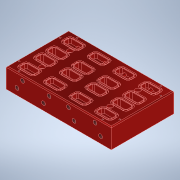
# Autodesk Inventor part: UNLHEP-14-01-P-004_ChuckForGantry
Saved by Autodesk Inventor 2022 (Build 260153000, 153)
## iProperties
Created: 2014-01-09
Part Number: UNLHEP-14-01-P-004_ChuckForGantry
Material: Aluminum, Anodized Red
Document SubType Name: Modeling
Designer: Frank Meier
Density: 2.7 g/cm^3
Project: UNL Pixel Phase I
Mass: 2699.72 g
Surface Area: 1115.91 cm^2
Volume: 999.896 cm^3
Appearance: Anodized - Red
Author: Frank Meier
Revision Number: 00
Autodesk Inventor part; units mm, degrees
ref_plane "YZ Plane" through (0, 0, 0) normal (1, 0, 0) x (0, 1, 0)
ref_plane "XZ Plane" through (0, 0, 0) normal (0, 1, 0) x (-1, 0, 0)
ref_plane "XY Plane" through (0, 0, 0) normal (0, 0, 1) x (1, 0, 0)
sketch "Skizze1" plane through (0, 0, 0) normal (0, 0, 1) x (1, 0, 0)
  line L0 (-117.475, -69.85) -> (117.475, -69.85)
  line L1 (117.475, -69.85) -> (117.475, 69.85)
  line L2 (117.475, 69.85) -> (-117.475, 69.85)
  line L3 (-117.475, 69.85) -> (-117.475, -69.85)
  line L4 (-117.475, -69.85) -> (117.475, 69.85) construction
  line L5 (117.475, -69.85) -> (-117.475, 69.85) construction
  point P0 (0, 0)
  dimension "d0" = 234.95
  dimension "d2" = 139.7
  constraints: 12 end point, 2 midpoint, 2 parallel, 1 horizontal, 1 perpendicular
  measures "d0" distance of L1.end L2.end
  measures "d2" distance of L0.end L1.end
extrude "Extrusion1" add sketch "Skizze1" along normal blind 44.45
chamfer "Fase1" distance 2 angle 45 4 edges at (0, -69.85, 44.45) (-117.475, 0, 44.45) (0, 69.85, 44.45) (117.475, 0, 44.45)
sketch "Alignment Holes" plane through (0, 0, 44.45) normal (0, 0, 1) x (1, 0, 0)
  line L0 (117.475, 69.85) -> (-117.475, 69.85) projected
  line L1 (117.475, -69.85) -> (117.475, 69.85) projected
  line L2 (-117.475, 69.85) -> (-117.475, -69.85) projected
  line L3 (-117.475, -69.85) -> (117.475, -69.85) projected
  point P0 (-112.475, 45.85)
  point P1 (-112.475, -45.85)
  point P2 (-93.475, -64.85)
  point P3 (-93.475, 64.85)
  point P4 (93.475, 64.85)
  point P5 (112.475, 45.85)
  point P6 (112.475, -45.85)
  point P7 (93.475, -64.85)
  dimension "d153" = 24
  dimension "d154" = 24
  dimension "d155" = 5
  dimension "d156" = 5
  dimension "d157" = 24
  dimension "d158" = 5
  dimension "d159" = 5
  dimension "d160" = 24
  dimension "d161" = 24
  dimension "d162" = 5
  dimension "d163" = 5
  dimension "d164" = 24
  dimension "d165" = 5
  dimension "d166" = 24
  dimension "d167" = 5
  dimension "d168" = 24
  measures "d153" distance from line of L0 point (-112.475, 45.85)
  measures "d154" distance from line of L3 point (-112.475, -45.85)
  measures "d155" distance from line of L2 point (-112.475, -45.85)
  measures "d156" distance from line of L3 point (-93.475, -64.85)
  measures "d157" distance from line of L2 point (-93.475, -64.85)
  measures "d158" distance from line of L2 point (-112.475, 45.85)
  measures "d159" distance from line of L0 point (-93.475, 64.85)
  measures "d160" distance from line of L2 point (-93.475, 64.85)
  measures "d161" distance from line of L1 point (93.475, 64.85)
  measures "d162" distance from line of L0 point (93.475, 64.85)
  measures "d163" distance from line of L1 point (112.475, 45.85)
  measures "d164" distance from line of L0 point (112.475, 45.85)
  measures "d165" distance from line of L1 point (112.475, -45.85)
  measures "d166" distance from line of L3 point (112.475, -45.85)
  measures "d167" distance from line of L3 point (93.475, -64.85)
  measures "d168" distance from line of L1 point (93.475, -64.85)
hole "Bohrung7" at (-112.475, 45.85, 44.45) at (-112.475, -45.85, 44.45) at (-93.475, -64.85, 44.45) at (-93.475, 64.85, 44.45) at (93.475, 64.85, 44.45) at (112.475, 45.85, 44.45) at (112.475, -45.85, 44.45) at (93.475, -64.85, 44.45) direction (0, 0, -1) diameter 3.242 depth 20 tip angle 118 thread size "M4x0.7" class "6H" standard "ISO Metric profile"
sketch "Wells" plane through (0, 0, 44.45) normal (0, 0, 1) x (1, 0, 0)
  line L0 (-97.975, 56.35) -> (-73.975, 56.35)
  line L1 (-70.975, 53.35) -> (-70.975, 44.35)
  line L2 (-73.975, 41.35) -> (-97.975, 41.35)
  line L3 (-100.975, 44.35) -> (-100.975, 53.35)
  circle A0 centre (-93.475, 64.85) radius 1.621 projected
  circle A1 centre (-112.475, 45.85) radius 1.621 projected
  arc A2 (-97.975, 56.35) -> (-100.975, 53.35) centre (-97.975, 53.35) ccw
  arc A3 (-70.975, 53.35) -> (-73.975, 56.35) centre (-73.975, 53.35) ccw
  arc A4 (-73.975, 41.35) -> (-70.975, 44.35) centre (-73.975, 44.35) ccw
  arc A5 (-100.975, 44.35) -> (-97.975, 41.35) centre (-97.975, 44.35) ccw
  arc A6 (-40.658, 56.35) -> (-43.658, 53.35) centre (-40.658, 53.35) ccw
  line L4 (-43.658, 44.35) -> (-43.658, 53.35)
  arc A7 (-43.658, 44.35) -> (-40.658, 41.35) centre (-40.658, 44.35) ccw
  line L5 (-40.658, 56.35) -> (-16.658, 56.35)
  arc A8 (-13.658, 53.35) -> (-16.658, 56.35) centre (-16.658, 53.35) ccw
  line L6 (-13.658, 53.35) -> (-13.658, 44.35)
  line L7 (-16.658, 41.35) -> (-40.658, 41.35)
  arc A9 (-16.658, 41.35) -> (-13.658, 44.35) centre (-16.658, 44.35) ccw
  arc A10 (16.659, 56.35) -> (13.659, 53.35) centre (16.659, 53.35) ccw
  line L8 (13.659, 44.35) -> (13.659, 53.35)
  arc A11 (13.659, 44.35) -> (16.659, 41.35) centre (16.659, 44.35) ccw
  line L9 (16.659, 56.35) -> (40.659, 56.35)
  arc A12 (43.659, 53.35) -> (40.659, 56.35) centre (40.659, 53.35) ccw
  line L10 (43.659, 53.35) -> (43.659, 44.35)
  line L11 (40.659, 41.35) -> (16.659, 41.35)
  arc A13 (40.659, 41.35) -> (43.659, 44.35) centre (40.659, 44.35) ccw
  arc A14 (73.976, 56.35) -> (70.976, 53.35) centre (73.976, 53.35) ccw
  line L12 (70.976, 44.35) -> (70.976, 53.35)
  arc A15 (70.976, 44.35) -> (73.976, 41.35) centre (73.976, 44.35) ccw
  line L13 (73.976, 56.35) -> (97.976, 56.35)
  arc A16 (100.976, 53.35) -> (97.976, 56.35) centre (97.976, 53.35) ccw
  line L14 (100.976, 53.35) -> (100.976, 44.35)
  line L15 (97.976, 41.35) -> (73.976, 41.35)
  arc A17 (97.976, 41.35) -> (100.976, 44.35) centre (97.976, 44.35) ccw
  arc A18 (-97.975, 20.784) -> (-100.975, 17.784) centre (-97.975, 17.784) ccw
  line L16 (-100.975, 8.784) -> (-100.975, 17.784)
  arc A19 (-100.975, 8.784) -> (-97.975, 5.784) centre (-97.975, 8.784) ccw
  line L17 (-97.975, 20.784) -> (-73.975, 20.784)
  arc A20 (-70.975, 17.784) -> (-73.975, 20.784) centre (-73.975, 17.784) ccw
  line L18 (-70.975, 17.784) -> (-70.975, 8.784)
  line L19 (-73.975, 5.784) -> (-97.975, 5.784)
  arc A21 (-73.975, 5.784) -> (-70.975, 8.784) centre (-73.975, 8.784) ccw
  arc A22 (-40.658, 20.784) -> (-43.658, 17.784) centre (-40.658, 17.784) ccw
  line L20 (-43.658, 8.784) -> (-43.658, 17.784)
  arc A23 (-43.658, 8.784) -> (-40.658, 5.784) centre (-40.658, 8.784) ccw
  line L21 (-40.658, 20.784) -> (-16.658, 20.784)
  arc A24 (-13.658, 17.784) -> (-16.658, 20.784) centre (-16.658, 17.784) ccw
  line L22 (-13.658, 17.784) -> (-13.658, 8.784)
  line L23 (-16.658, 5.784) -> (-40.658, 5.784)
  arc A25 (-16.658, 5.784) -> (-13.658, 8.784) centre (-16.658, 8.784) ccw
  arc A26 (16.659, 20.784) -> (13.659, 17.784) centre (16.659, 17.784) ccw
  line L24 (13.659, 8.784) -> (13.659, 17.784)
  arc A27 (13.659, 8.784) -> (16.659, 5.784) centre (16.659, 8.784) ccw
  line L25 (16.659, 20.784) -> (40.659, 20.784)
  arc A28 (43.659, 17.784) -> (40.659, 20.784) centre (40.659, 17.784) ccw
  line L26 (43.659, 17.784) -> (43.659, 8.784)
  line L27 (40.659, 5.784) -> (16.659, 5.784)
  arc A29 (40.659, 5.784) -> (43.659, 8.784) centre (40.659, 8.784) ccw
  arc A30 (73.976, 20.784) -> (70.976, 17.784) centre (73.976, 17.784) ccw
  line L28 (70.976, 8.784) -> (70.976, 17.784)
  arc A31 (70.976, 8.784) -> (73.976, 5.784) centre (73.976, 8.784) ccw
  line L29 (73.976, 20.784) -> (97.976, 20.784)
  arc A32 (100.976, 17.784) -> (97.976, 20.784) centre (97.976, 17.784) ccw
  line L30 (100.976, 17.784) -> (100.976, 8.784)
  line L31 (97.976, 5.784) -> (73.976, 5.784)
  arc A33 (97.976, 5.784) -> (100.976, 8.784) centre (97.976, 8.784) ccw
  circle A34 centre (-93.475, -64.85) radius 1.621 projected
  circle A35 centre (112.475, 45.85) radius 1.621 projected
  line L32 (97.975, -56.35) -> (73.975, -56.35)
  line L33 (70.975, -53.35) -> (70.975, -44.35)
  line L34 (73.975, -41.35) -> (97.975, -41.35)
  line L35 (100.975, -44.35) -> (100.975, -53.35)
  circle A36 centre (112.475, -45.85) radius 1.621 projected
  circle A37 centre (93.475, -64.85) radius 1.621 projected
  arc A38 (73.975, -41.35) -> (70.975, -44.35) centre (73.975, -44.35) ccw
  arc A39 (70.975, -53.35) -> (73.975, -56.35) centre (73.975, -53.35) ccw
  arc A40 (97.975, -56.35) -> (100.975, -53.35) centre (97.975, -53.35) ccw
  arc A41 (100.975, -44.35) -> (97.975, -41.35) centre (97.975, -44.35) ccw
  arc A42 (43.658, -44.35) -> (40.658, -41.35) centre (40.658, -44.35) ccw
  line L36 (16.658, -41.35) -> (40.658, -41.35)
  line L37 (43.658, -44.35) -> (43.658, -53.35)
  arc A43 (40.658, -56.35) -> (43.658, -53.35) centre (40.658, -53.35) ccw
  line L38 (40.658, -56.35) -> (16.658, -56.35)
  arc A44 (16.658, -41.35) -> (13.658, -44.35) centre (16.658, -44.35) ccw
  arc A45 (13.658, -53.35) -> (16.658, -56.35) centre (16.658, -53.35) ccw
  line L39 (13.658, -53.35) -> (13.658, -44.35)
  arc A46 (-13.659, -44.35) -> (-16.659, -41.35) centre (-16.659, -44.35) ccw
  line L40 (-40.659, -41.35) -> (-16.659, -41.35)
  line L41 (-13.659, -44.35) -> (-13.659, -53.35)
  arc A47 (-16.659, -56.35) -> (-13.659, -53.35) centre (-16.659, -53.35) ccw
  line L42 (-16.659, -56.35) -> (-40.659, -56.35)
  arc A48 (-40.659, -41.35) -> (-43.659, -44.35) centre (-40.659, -44.35) ccw
  arc A49 (-43.659, -53.35) -> (-40.659, -56.35) centre (-40.659, -53.35) ccw
  line L43 (-43.659, -53.35) -> (-43.659, -44.35)
  arc A50 (-70.976, -44.35) -> (-73.976, -41.35) centre (-73.976, -44.35) ccw
  line L44 (-97.976, -41.35) -> (-73.976, -41.35)
  line L45 (-70.976, -44.35) -> (-70.976, -53.35)
  arc A51 (-73.976, -56.35) -> (-70.976, -53.35) centre (-73.976, -53.35) ccw
  line L46 (-73.976, -56.35) -> (-97.976, -56.35)
  arc A52 (-97.976, -41.35) -> (-100.976, -44.35) centre (-97.976, -44.35) ccw
  arc A53 (-100.976, -53.35) -> (-97.976, -56.35) centre (-97.976, -53.35) ccw
  line L47 (-100.976, -53.35) -> (-100.976, -44.35)
  arc A54 (100.975, -8.784) -> (97.975, -5.784) centre (97.975, -8.784) ccw
  line L48 (73.975, -5.784) -> (97.975, -5.784)
  line L49 (100.975, -8.784) -> (100.975, -17.784)
  arc A55 (97.975, -20.784) -> (100.975, -17.784) centre (97.975, -17.784) ccw
  line L50 (97.975, -20.784) -> (73.975, -20.784)
  arc A56 (73.975, -5.784) -> (70.975, -8.784) centre (73.975, -8.784) ccw
  arc A57 (70.975, -17.784) -> (73.975, -20.784) centre (73.975, -17.784) ccw
  line L51 (70.975, -17.784) -> (70.975, -8.784)
  arc A58 (43.658, -8.784) -> (40.658, -5.784) centre (40.658, -8.784) ccw
  line L52 (16.658, -5.784) -> (40.658, -5.784)
  line L53 (43.658, -8.784) -> (43.658, -17.784)
  arc A59 (40.658, -20.784) -> (43.658, -17.784) centre (40.658, -17.784) ccw
  line L54 (40.658, -20.784) -> (16.658, -20.784)
  arc A60 (16.658, -5.784) -> (13.658, -8.784) centre (16.658, -8.784) ccw
  arc A61 (13.658, -17.784) -> (16.658, -20.784) centre (16.658, -17.784) ccw
  line L55 (13.658, -17.784) -> (13.658, -8.784)
  arc A62 (-13.659, -8.784) -> (-16.659, -5.784) centre (-16.659, -8.784) ccw
  line L56 (-40.659, -5.784) -> (-16.659, -5.784)
  line L57 (-13.659, -8.784) -> (-13.659, -17.784)
  arc A63 (-16.659, -20.784) -> (-13.659, -17.784) centre (-16.659, -17.784) ccw
  line L58 (-16.659, -20.784) -> (-40.659, -20.784)
  arc A64 (-40.659, -5.784) -> (-43.659, -8.784) centre (-40.659, -8.784) ccw
  arc A65 (-43.659, -17.784) -> (-40.659, -20.784) centre (-40.659, -17.784) ccw
  line L59 (-43.659, -17.784) -> (-43.659, -8.784)
  arc A66 (-70.976, -8.784) -> (-73.976, -5.784) centre (-73.976, -8.784) ccw
  line L60 (-97.976, -5.784) -> (-73.976, -5.784)
  line L61 (-70.976, -8.784) -> (-70.976, -17.784)
  arc A67 (-73.976, -20.784) -> (-70.976, -17.784) centre (-73.976, -17.784) ccw
  line L62 (-73.976, -20.784) -> (-97.976, -20.784)
  arc A68 (-97.976, -5.784) -> (-100.976, -8.784) centre (-97.976, -8.784) ccw
  arc A69 (-100.976, -17.784) -> (-97.976, -20.784) centre (-97.976, -17.784) ccw
  line L63 (-100.976, -17.784) -> (-100.976, -8.784)
  point P0 (0, 0)
  point P1 (-70.975, 41.35)
  point P2 (-70.975, 56.35)
  point P3 (-100.975, 41.35)
  point P4 (-43.658, 41.35)
  point P5 (-13.658, 56.35)
  point P6 (-13.658, 41.35)
  point P7 (13.659, 41.35)
  point P8 (43.659, 56.35)
  point P9 (43.659, 41.35)
  point P10 (70.976, 41.35)
  point P11 (100.976, 56.35)
  point P12 (100.976, 41.35)
  point P13 (-100.975, 5.784)
  point P14 (-70.975, 20.784)
  point P15 (-70.975, 5.784)
  point P16 (-43.658, 5.784)
  point P17 (-13.658, 20.784)
  point P18 (-13.658, 5.784)
  point P19 (13.659, 5.784)
  point P20 (43.659, 20.784)
  point P21 (43.659, 5.784)
  point P22 (70.976, 5.784)
  point P23 (100.976, 20.784)
  point P24 (100.976, 5.784)
  point P25 (100.975, -56.35)
  point P26 (70.975, -56.35)
  point P27 (100.975, -41.35)
  point P28 (43.658, -41.35)
  point P29 (43.658, -56.35)
  point P30 (13.658, -56.35)
  point P31 (-13.659, -41.35)
  point P32 (-13.659, -56.35)
  point P33 (-43.659, -56.35)
  point P34 (-70.976, -41.35)
  point P35 (-70.976, -56.35)
  point P36 (-100.976, -56.35)
  point P37 (100.975, -5.784)
  point P38 (100.975, -20.784)
  point P39 (70.975, -20.784)
  point P40 (43.658, -5.784)
  point P41 (43.658, -20.784)
  point P42 (13.658, -20.784)
  point P43 (-13.659, -5.784)
  point P44 (-13.659, -20.784)
  point P45 (-43.659, -20.784)
  point P46 (-70.976, -5.784)
  point P47 (-70.976, -20.784)
  point P48 (-100.976, -20.784)
  dimension "d259" = 30
  dimension "d260" = 15
  dimension "d261" = 8.5
  dimension "d262" = 11.5
  dimension "d266" = 3
  dimension "d269" = 57.317
  dimension "d272" = 35.566
  dimension "d276" = 11.499
  dimension "d410" = 11.5
  dimension "d411" = 8.5
  dimension "d412" = 15
  dimension "d413" = 30
  dimension "d414" = 3
  dimension "d417" = 57.317
  dimension "d420" = 35.566
  constraints: 128 end point, 128 point on circle, 96 point on line, 64 centre point, 16 tangent, 6 equal radius, 4 collinear, 4 horizontal, 4 parallel, 2 perpendicular, 2 vertical, 318 other
  measures "d259" distance of point (-70.975, 41.35) point (-100.975, 41.35)
  measures "d260" distance of point (-70.975, 56.35) point (-70.975, 41.35)
  measures "d261" distance from line of L0 A0.centre
  measures "d262" distance from line of L3 A1.centre
  measures "d266" radius of A2
  measures "d269" distance of L3.end L4.end
  measures "d272" distance of L3.end L16.end
  measures "d276" distance from line of L14 A35.centre
  measures "d410" distance from line of L35 A36.centre
  measures "d411" distance from line of A37.centre L32
  measures "d412" distance of point (100.975, -41.35) point (100.975, -56.35)
  measures "d413" distance of point (100.975, -56.35) point (70.975, -56.35)
  measures "d414" radius of A38
  measures "d417" distance of point (100.975, -41.35) point (43.658, -41.35)
  measures "d420" distance of point (100.975, -41.35) point (100.975, -5.784)
extrude "Extrusion6" cut sketch "Wells" against normal blind 10 contours L0 A3 L1 A4 L2 A5 L3 A2 | L5 A8 L6 A9 L7 A7 L4 A6 | L9 A12 L10 A13 L11 A11 L8 A10 | L13 A16 L14 A17 L15 A15 L12 A14 | L32 A39 L33 A38 L34 A41 L35 A40 | L37 A43 L38 A45 L39 A44 L36 A42 | L41 A47 L42 A49 L43 A48 L40 A46 | L45 A51 L46 A53 L47 A52 L44 A50
extrude "Extrusion7" cut sketch "Wells" against normal blind 30 contours L17 A20 L18 A21 L19 A19 L16 A18 | L21 A24 L22 A25 L23 A23 L20 A22 | L25 A28 L26 A29 L27 A27 L24 A26 | L29 A32 L30 A33 L31 A31 L28 A30 | L49 A55 L50 A57 L51 A56 L48 A54 | L53 A59 L54 A61 L55 A60 L52 A58 | L57 A63 L58 A65 L59 A64 L56 A62 | L61 A67 L62 A69 L63 A68 L60 A66
sketch "Sketch17" plane through (-117.475, -69.85, 0) normal (0, -1, 0) x (1, 0, 0)
  line L0 (232.95, 44.45) -> (2, 44.45) projected
  line L1 (46.499, 44.45) -> (46.499, 14.45) projected
  line L2 (188.45, 44.45) -> (188.45, 14.45) projected
  point P0 (117.475, 0)
  point P1 (36.499, 34.45)
  point P2 (23.999, 14.45)
  point P3 (83.316, 14.45)
  point P4 (95.816, 34.45)
  point P5 (198.45, 34.45)
  point P6 (210.95, 14.45)
  point P7 (139.133, 34.45)
  point P8 (151.633, 14.45)
  dimension "d283" = 10
  dimension "d286" = 59.317
  dimension "d328" = 59.317
  dimension "d443" = 10
  dimension "d444" = 10
  dimension "d450" = 20
  dimension "d451" = 12.5
  dimension "d452" = 12.5
  constraints: 2 horizontal, 2 horizontal alignment, 4 other
  measures "d283" distance from line of L0 point (36.499, 34.45)
  measures "d286" distance of point (23.999, 14.45) point (83.316, 14.45)
  measures "d328" distance of point (198.45, 34.45) point (139.133, 34.45)
  measures "d443" distance from line of L1 point (36.499, 34.45)
  measures "d444" distance from line of L2 point (198.45, 34.45)
  measures "d450" vertical distance of point (23.999, 14.45) point (36.499, 34.45)
  measures "d451" horizontal distance of point (23.999, 14.45) point (36.499, 34.45)
  measures "d452" horizontal distance of point (210.95, 14.45) point (198.45, 34.45)
hole "Hole12" at (-80.976, -69.85, 34.45) at (-21.659, -69.85, 34.45) at (21.658, -69.85, 34.45) at (80.975, -69.85, 34.45) direction (0, 1, 0) diameter 7.9502 depth 20 tip angle 118 taper from width 8.7366 to width 8.304 over 6.924 thread size "1/8" designation "1/8 - 27 NPT" standard "NPT"
hole "Hole13" at (-93.476, -69.85, 14.45) at (-34.159, -69.85, 14.45) at (34.158, -69.85, 14.45) at (93.475, -69.85, 14.45) direction (0, 1, 0) diameter 7.9502 depth 55 tip angle 118 taper from width 8.7366 to width 8.304 over 6.924 thread size "1/8" designation "1/8 - 27 NPT" standard "NPT"
sketch "Sketch19" plane through (-117.475, 69.85, 0) normal (0, 1, 0) x (1, 0, 0)
  arc A0 (40.4741, -34.45) -> (32.5239, -34.45) centre (36.499, -34.45) ccw projected
  circle A1 centre (95.816, -34.45) radius 3.9751 projected
  circle A2 centre (139.133, -34.45) radius 4.152 projected
  circle A3 centre (210.95, -14.45) radius 4.3684
  circle A4 centre (198.45, -34.45) radius 3.9751 projected
  line L0 (210.95, -23.476) -> (212.571, -24.45) projected
  line L1 (210.95, -23.476) -> (209.329, -24.45) projected
  point P0 (117.475, 0)
  point P1 (23.999, -14.5362)
  point P2 (83.316, -14.45)
  point P3 (95.816, -14.45)
  point P4 (151.633, -14.393)
  dimension "d446" = 12.5
  dimension "d447" = 12.5
  dimension "d448" = 12.5
  dimension "d449" = 12.5
  constraints: 5 coincident, 1 centre point, 1 vertical alignment
  measures "d446" horizontal distance of point (210.95, -14.45) point (198.45, -34.45)
  measures "d447" horizontal distance of point (151.633, -14.393) point (139.133, -34.45)
  measures "d448" horizontal distance of A1.centre point (83.316, -14.45)
  measures "d449" horizontal distance of point (23.999, -14.536) A0.centre
hole "Hole15" at (93.475, 69.85, 14.45) at (-34.159, 69.85, 14.45) at (-93.476, 69.85, 14.5362) at (34.158, 69.85, 14.393) direction (0, -1, 0) diameter 7.9502 depth 55 tip angle 118 taper from width 8.7366 to width 8.304 over 6.924 thread size "1/8" designation "1/8 - 27 NPT" standard "NPT"
hole "Hole16" at (-80.976, 69.85, 34.45) at (-21.659, 69.85, 34.45) at (21.658, 69.85, 34.45) at (80.975, 69.85, 34.45) direction (0, -1, 0) diameter 7.9502 depth 20 tip angle 118 taper from width 8.7366 to width 8.304 over 6.924 thread size "1/8" designation "1/8 - 27 NPT" standard "NPT"
sketch "Sketch22" plane through (0, 0, 44.45) normal (0, 0, 1) x (1, 0, 0)
  point P0 (0, 0)
  point P1 (76.2, -31)
  point P2 (-76.2, -31)
  point P3 (-76.2, 31)
  point P4 (76.2, 31)
  dimension "d382" = 76.2
  dimension "d383" = 152.4
  dimension "d384" = 31
  dimension "d385" = 62
  constraints: 2 horizontal alignment, 2 vertical alignment
  measures "d382" horizontal distance of point (76.2, -31) point (0, 0)
  measures "d383" distance of point (76.2, -31) point (-76.2, -31)
  measures "d384" vertical distance of point (76.2, -31) point (0, 0)
  measures "d385" distance of point (76.2, -31) point (76.2, 31)
hole "Hole18" at (76.2, -31, 44.45) at (-76.2, -31, 44.45) at (-76.2, 31, 44.45) at (76.2, 31, 44.45) direction (0, 0, -1) diameter 6.7564 end through all counterbore diameter 11.1252 counterbore depth 6.35 clearance for "Socket Head Cap Screw" size "1/4" standard "Ansi Unified Screw Threads"
sketch "Seal Seating" plane through (0, 0, 44.45) normal (0, 0, 1) x (1, 0, 0)
  line L0 (-97.975, 56.35) -> (-73.975, 56.35) projected
  line L1 (-70.975, 53.35) -> (-70.975, 44.35) projected
  line L2 (-100.975, 44.35) -> (-100.975, 53.35) projected
  line L3 (-73.975, 41.35) -> (-97.975, 41.35) projected
  arc A0 (-97.975, 56.35) -> (-100.975, 53.35) centre (-97.975, 53.35) ccw
  arc A1 (-97.975, 57.62) -> (-102.245, 53.35) centre (-97.975, 53.35) ccw
  arc A2 (-70.975, 53.35) -> (-73.975, 56.35) centre (-73.975, 53.35) ccw
  arc A3 (-73.975, 41.35) -> (-70.975, 44.35) centre (-73.975, 44.35) ccw
  arc A4 (-100.975, 44.35) -> (-97.975, 41.35) centre (-97.975, 44.35) ccw
  line L4 (-73.975, 41.35) -> (-97.975, 41.35)
  line L5 (-100.975, 44.35) -> (-100.975, 53.35)
  line L6 (-97.975, 56.35) -> (-73.975, 56.35)
  line L7 (-70.975, 53.35) -> (-70.975, 44.35)
  arc A5 (-69.705, 53.35) -> (-73.975, 57.62) centre (-73.975, 53.35) ccw
  arc A6 (-73.975, 40.08) -> (-69.705, 44.35) centre (-73.975, 44.35) ccw
  arc A7 (-102.245, 44.35) -> (-97.975, 40.08) centre (-97.975, 44.35) ccw
  line L8 (-97.975, 57.62) -> (-73.975, 57.62)
  line L9 (-69.705, 53.35) -> (-69.705, 44.35)
  line L10 (-73.975, 41.35) -> (-97.975, 41.35)
  line L11 (-73.975, 40.08) -> (-97.975, 40.08)
  line L12 (-102.245, 44.35) -> (-102.245, 53.35)
  arc A8 (-97.975, 60.795) -> (-105.42, 53.35) centre (-97.975, 53.35) ccw
  arc A9 (-66.53, 53.35) -> (-73.975, 60.795) centre (-73.975, 53.35) ccw
  arc A10 (-73.975, 36.905) -> (-66.53, 44.35) centre (-73.975, 44.35) ccw
  arc A11 (-105.42, 44.35) -> (-97.975, 36.905) centre (-97.975, 44.35) ccw
  line L13 (-105.42, 44.35) -> (-105.42, 53.35)
  line L14 (-97.975, 60.795) -> (-73.975, 60.795)
  line L15 (-66.53, 53.35) -> (-66.53, 44.35)
  line L16 (-73.975, 36.905) -> (-97.975, 36.905)
  arc A12 (-70.975, 53.35) -> (-73.975, 56.35) centre (-73.975, 53.35) ccw projected
  arc A13 (-97.975, 56.35) -> (-100.975, 53.35) centre (-97.975, 53.35) ccw projected
  arc A14 (-100.975, 44.35) -> (-97.975, 41.35) centre (-97.975, 44.35) ccw projected
  arc A15 (-73.975, 41.35) -> (-70.975, 44.35) centre (-73.975, 44.35) ccw projected
  arc A16 (-16.6472, 41.35) -> (-13.6472, 44.35) centre (-16.6472, 44.35) ccw
  arc A17 (-16.6472, 40.08) -> (-12.3772, 44.35) centre (-16.6472, 44.35) ccw
  arc A18 (-16.6472, 36.905) -> (-9.2022, 44.35) centre (-16.6472, 44.35) ccw
  arc A19 (-44.9172, 44.35) -> (-40.6472, 40.08) centre (-40.6472, 44.35) ccw
  arc A20 (-48.0922, 44.35) -> (-40.6472, 36.905) centre (-40.6472, 44.35) ccw
  line L17 (-13.6472, 53.35) -> (-13.6472, 44.35)
  line L18 (-12.3772, 53.35) -> (-12.3772, 44.35)
  line L19 (-9.2022, 53.35) -> (-9.2022, 44.35)
  arc A21 (-13.6472, 53.35) -> (-16.6472, 56.35) centre (-16.6472, 53.35) ccw
  arc A22 (-12.3772, 53.35) -> (-16.6472, 57.62) centre (-16.6472, 53.35) ccw
  arc A23 (-9.2022, 53.35) -> (-16.6472, 60.795) centre (-16.6472, 53.35) ccw
  arc A24 (-40.6472, 56.35) -> (-43.6472, 53.35) centre (-40.6472, 53.35) ccw
  arc A25 (-43.6472, 44.35) -> (-40.6472, 41.35) centre (-40.6472, 44.35) ccw
  line L20 (-43.6472, 44.35) -> (-43.6472, 53.35)
  line L21 (-48.0922, 44.35) -> (-48.0922, 53.35)
  line L22 (-44.9172, 44.35) -> (-44.9172, 53.35)
  arc A26 (-40.6472, 60.795) -> (-48.0922, 53.35) centre (-40.6472, 53.35) ccw
  arc A27 (-40.6472, 57.62) -> (-44.9172, 53.35) centre (-40.6472, 53.35) ccw
  line L23 (-16.6472, 36.905) -> (-40.6472, 36.905)
  line L24 (-16.6472, 40.08) -> (-40.6472, 40.08)
  line L25 (-16.6472, 41.35) -> (-40.6472, 41.35)
  line L26 (-16.6472, 41.35) -> (-40.6472, 41.35)
  line L27 (-40.6472, 56.35) -> (-16.6472, 56.35)
  line L28 (-40.6472, 57.62) -> (-16.6472, 57.62)
  line L29 (-40.6472, 60.795) -> (-16.6472, 60.795)
  arc A28 (40.6806, 41.35) -> (43.6806, 44.35) centre (40.6806, 44.35) ccw
  arc A29 (40.6806, 40.08) -> (44.9506, 44.35) centre (40.6806, 44.35) ccw
  arc A30 (40.6806, 36.905) -> (48.1256, 44.35) centre (40.6806, 44.35) ccw
  arc A31 (12.4106, 44.35) -> (16.6806, 40.08) centre (16.6806, 44.35) ccw
  arc A32 (9.2356, 44.35) -> (16.6806, 36.905) centre (16.6806, 44.35) ccw
  line L30 (43.6806, 53.35) -> (43.6806, 44.35)
  line L31 (44.9506, 53.35) -> (44.9506, 44.35)
  line L32 (48.1256, 53.35) -> (48.1256, 44.35)
  arc A33 (43.6806, 53.35) -> (40.6806, 56.35) centre (40.6806, 53.35) ccw
  arc A34 (44.9506, 53.35) -> (40.6806, 57.62) centre (40.6806, 53.35) ccw
  arc A35 (48.1256, 53.35) -> (40.6806, 60.795) centre (40.6806, 53.35) ccw
  arc A36 (16.6806, 56.35) -> (13.6806, 53.35) centre (16.6806, 53.35) ccw
  arc A37 (13.6806, 44.35) -> (16.6806, 41.35) centre (16.6806, 44.35) ccw
  line L33 (13.6806, 44.35) -> (13.6806, 53.35)
  line L34 (9.2356, 44.35) -> (9.2356, 53.35)
  line L35 (12.4106, 44.35) -> (12.4106, 53.35)
  arc A38 (16.6806, 60.795) -> (9.2356, 53.35) centre (16.6806, 53.35) ccw
  arc A39 (16.6806, 57.62) -> (12.4106, 53.35) centre (16.6806, 53.35) ccw
  line L36 (40.6806, 36.905) -> (16.6806, 36.905)
  line L37 (40.6806, 40.08) -> (16.6806, 40.08)
  line L38 (40.6806, 41.35) -> (16.6806, 41.35)
  line L39 (40.6806, 41.35) -> (16.6806, 41.35)
  line L40 (16.6806, 56.35) -> (40.6806, 56.35)
  line L41 (16.6806, 57.62) -> (40.6806, 57.62)
  line L42 (16.6806, 60.795) -> (40.6806, 60.795)
  arc A40 (98.0084, 41.35) -> (101.0084, 44.35) centre (98.0084, 44.35) ccw
  arc A41 (98.0084, 40.08) -> (102.2784, 44.35) centre (98.0084, 44.35) ccw
  arc A42 (98.0084, 36.905) -> (105.4534, 44.35) centre (98.0084, 44.35) ccw
  arc A43 (69.7384, 44.35) -> (74.0084, 40.08) centre (74.0084, 44.35) ccw
  arc A44 (66.5634, 44.35) -> (74.0084, 36.905) centre (74.0084, 44.35) ccw
  line L43 (101.0084, 53.35) -> (101.0084, 44.35)
  line L44 (102.2784, 53.35) -> (102.2784, 44.35)
  line L45 (105.4534, 53.35) -> (105.4534, 44.35)
  arc A45 (101.0084, 53.35) -> (98.0084, 56.35) centre (98.0084, 53.35) ccw
  arc A46 (102.2784, 53.35) -> (98.0084, 57.62) centre (98.0084, 53.35) ccw
  arc A47 (105.4534, 53.35) -> (98.0084, 60.795) centre (98.0084, 53.35) ccw
  arc A48 (74.0084, 56.35) -> (71.0084, 53.35) centre (74.0084, 53.35) ccw
  arc A49 (71.0084, 44.35) -> (74.0084, 41.35) centre (74.0084, 44.35) ccw
  line L46 (71.0084, 44.35) -> (71.0084, 53.35)
  line L47 (66.5634, 44.35) -> (66.5634, 53.35)
  line L48 (69.7384, 44.35) -> (69.7384, 53.35)
  arc A50 (74.0084, 60.795) -> (66.5634, 53.35) centre (74.0084, 53.35) ccw
  arc A51 (74.0084, 57.62) -> (69.7384, 53.35) centre (74.0084, 53.35) ccw
  line L49 (98.0084, 36.905) -> (74.0084, 36.905)
  line L50 (98.0084, 40.08) -> (74.0084, 40.08)
  line L51 (98.0084, 41.35) -> (74.0084, 41.35)
  line L52 (98.0084, 41.35) -> (74.0084, 41.35)
  line L53 (74.0084, 56.35) -> (98.0084, 56.35)
  line L54 (74.0084, 57.62) -> (98.0084, 57.62)
  line L55 (74.0084, 60.795) -> (98.0084, 60.795)
  arc A52 (-73.975, 5.79) -> (-70.975, 8.79) centre (-73.975, 8.79) ccw
  arc A53 (-73.975, 4.52) -> (-69.705, 8.79) centre (-73.975, 8.79) ccw
  arc A54 (-73.975, 1.345) -> (-66.53, 8.79) centre (-73.975, 8.79) ccw
  arc A55 (-102.245, 8.79) -> (-97.975, 4.52) centre (-97.975, 8.79) ccw
  arc A56 (-105.42, 8.79) -> (-97.975, 1.345) centre (-97.975, 8.79) ccw
  line L56 (-70.975, 17.79) -> (-70.975, 8.79)
  line L57 (-69.705, 17.79) -> (-69.705, 8.79)
  line L58 (-66.53, 17.79) -> (-66.53, 8.79)
  arc A57 (-70.975, 17.79) -> (-73.975, 20.79) centre (-73.975, 17.79) ccw
  arc A58 (-69.705, 17.79) -> (-73.975, 22.06) centre (-73.975, 17.79) ccw
  arc A59 (-66.53, 17.79) -> (-73.975, 25.235) centre (-73.975, 17.79) ccw
  arc A60 (-97.975, 20.79) -> (-100.975, 17.79) centre (-97.975, 17.79) ccw
  arc A61 (-100.975, 8.79) -> (-97.975, 5.79) centre (-97.975, 8.79) ccw
  line L59 (-100.975, 8.79) -> (-100.975, 17.79)
  line L60 (-105.42, 8.79) -> (-105.42, 17.79)
  line L61 (-102.245, 8.79) -> (-102.245, 17.79)
  arc A62 (-97.975, 25.235) -> (-105.42, 17.79) centre (-97.975, 17.79) ccw
  arc A63 (-97.975, 22.06) -> (-102.245, 17.79) centre (-97.975, 17.79) ccw
  line L62 (-73.975, 1.345) -> (-97.975, 1.345)
  line L63 (-73.975, 4.52) -> (-97.975, 4.52)
  line L64 (-73.975, 5.79) -> (-97.975, 5.79)
  line L65 (-73.975, 5.79) -> (-97.975, 5.79)
  line L66 (-97.975, 20.79) -> (-73.975, 20.79)
  line L67 (-97.975, 22.06) -> (-73.975, 22.06)
  line L68 (-97.975, 25.235) -> (-73.975, 25.235)
  arc A64 (-16.6472, 5.79) -> (-13.6472, 8.79) centre (-16.6472, 8.79) ccw
  arc A65 (-16.6472, 4.52) -> (-12.3772, 8.79) centre (-16.6472, 8.79) ccw
  arc A66 (-16.6472, 1.345) -> (-9.2022, 8.79) centre (-16.6472, 8.79) ccw
  arc A67 (-44.9172, 8.79) -> (-40.6472, 4.52) centre (-40.6472, 8.79) ccw
  arc A68 (-48.0922, 8.79) -> (-40.6472, 1.345) centre (-40.6472, 8.79) ccw
  line L69 (-13.6472, 17.79) -> (-13.6472, 8.79)
  line L70 (-12.3772, 17.79) -> (-12.3772, 8.79)
  line L71 (-9.2022, 17.79) -> (-9.2022, 8.79)
  arc A69 (-13.6472, 17.79) -> (-16.6472, 20.79) centre (-16.6472, 17.79) ccw
  arc A70 (-12.3772, 17.79) -> (-16.6472, 22.06) centre (-16.6472, 17.79) ccw
  arc A71 (-9.2022, 17.79) -> (-16.6472, 25.235) centre (-16.6472, 17.79) ccw
  arc A72 (-40.6472, 20.79) -> (-43.6472, 17.79) centre (-40.6472, 17.79) ccw
  arc A73 (-43.6472, 8.79) -> (-40.6472, 5.79) centre (-40.6472, 8.79) ccw
  line L72 (-43.6472, 8.79) -> (-43.6472, 17.79)
  line L73 (-48.0922, 8.79) -> (-48.0922, 17.79)
  line L74 (-44.9172, 8.79) -> (-44.9172, 17.79)
  arc A74 (-40.6472, 25.235) -> (-48.0922, 17.79) centre (-40.6472, 17.79) ccw
  arc A75 (-40.6472, 22.06) -> (-44.9172, 17.79) centre (-40.6472, 17.79) ccw
  line L75 (-16.6472, 1.345) -> (-40.6472, 1.345)
  line L76 (-16.6472, 4.52) -> (-40.6472, 4.52)
  line L77 (-16.6472, 5.79) -> (-40.6472, 5.79)
  line L78 (-16.6472, 5.79) -> (-40.6472, 5.79)
  line L79 (-40.6472, 20.79) -> (-16.6472, 20.79)
  line L80 (-40.6472, 22.06) -> (-16.6472, 22.06)
  line L81 (-40.6472, 25.235) -> (-16.6472, 25.235)
  arc A76 (40.6806, 5.79) -> (43.6806, 8.79) centre (40.6806, 8.79) ccw
  arc A77 (40.6806, 4.52) -> (44.9506, 8.79) centre (40.6806, 8.79) ccw
  arc A78 (40.6806, 1.345) -> (48.1256, 8.79) centre (40.6806, 8.79) ccw
  arc A79 (12.4106, 8.79) -> (16.6806, 4.52) centre (16.6806, 8.79) ccw
  arc A80 (9.2356, 8.79) -> (16.6806, 1.345) centre (16.6806, 8.79) ccw
  line L82 (43.6806, 17.79) -> (43.6806, 8.79)
  line L83 (44.9506, 17.79) -> (44.9506, 8.79)
  line L84 (48.1256, 17.79) -> (48.1256, 8.79)
  arc A81 (43.6806, 17.79) -> (40.6806, 20.79) centre (40.6806, 17.79) ccw
  arc A82 (44.9506, 17.79) -> (40.6806, 22.06) centre (40.6806, 17.79) ccw
  arc A83 (48.1256, 17.79) -> (40.6806, 25.235) centre (40.6806, 17.79) ccw
  arc A84 (16.6806, 20.79) -> (13.6806, 17.79) centre (16.6806, 17.79) ccw
  arc A85 (13.6806, 8.79) -> (16.6806, 5.79) centre (16.6806, 8.79) ccw
  line L85 (13.6806, 8.79) -> (13.6806, 17.79)
  line L86 (9.2356, 8.79) -> (9.2356, 17.79)
  line L87 (12.4106, 8.79) -> (12.4106, 17.79)
  arc A86 (16.6806, 25.235) -> (9.2356, 17.79) centre (16.6806, 17.79) ccw
  arc A87 (16.6806, 22.06) -> (12.4106, 17.79) centre (16.6806, 17.79) ccw
  line L88 (40.6806, 1.345) -> (16.6806, 1.345)
  line L89 (40.6806, 4.52) -> (16.6806, 4.52)
  line L90 (40.6806, 5.79) -> (16.6806, 5.79)
  line L91 (40.6806, 5.79) -> (16.6806, 5.79)
  line L92 (16.6806, 20.79) -> (40.6806, 20.79)
  line L93 (16.6806, 22.06) -> (40.6806, 22.06)
  line L94 (16.6806, 25.235) -> (40.6806, 25.235)
  arc A88 (98.0084, 5.79) -> (101.0084, 8.79) centre (98.0084, 8.79) ccw
  arc A89 (98.0084, 4.52) -> (102.2784, 8.79) centre (98.0084, 8.79) ccw
  arc A90 (98.0084, 1.345) -> (105.4534, 8.79) centre (98.0084, 8.79) ccw
  arc A91 (69.7384, 8.79) -> (74.0084, 4.52) centre (74.0084, 8.79) ccw
  arc A92 (66.5634, 8.79) -> (74.0084, 1.345) centre (74.0084, 8.79) ccw
  line L95 (101.0084, 17.79) -> (101.0084, 8.79)
  line L96 (102.2784, 17.79) -> (102.2784, 8.79)
  line L97 (105.4534, 17.79) -> (105.4534, 8.79)
  arc A93 (101.0084, 17.79) -> (98.0084, 20.79) centre (98.0084, 17.79) ccw
  arc A94 (102.2784, 17.79) -> (98.0084, 22.06) centre (98.0084, 17.79) ccw
  arc A95 (105.4534, 17.79) -> (98.0084, 25.235) centre (98.0084, 17.79) ccw
  arc A96 (74.0084, 20.79) -> (71.0084, 17.79) centre (74.0084, 17.79) ccw
  arc A97 (71.0084, 8.79) -> (74.0084, 5.79) centre (74.0084, 8.79) ccw
  line L98 (71.0084, 8.79) -> (71.0084, 17.79)
  line L99 (66.5634, 8.79) -> (66.5634, 17.79)
  line L100 (69.7384, 8.79) -> (69.7384, 17.79)
  arc A98 (74.0084, 25.235) -> (66.5634, 17.79) centre (74.0084, 17.79) ccw
  arc A99 (74.0084, 22.06) -> (69.7384, 17.79) centre (74.0084, 17.79) ccw
  line L101 (98.0084, 1.345) -> (74.0084, 1.345)
  line L102 (98.0084, 4.52) -> (74.0084, 4.52)
  line L103 (98.0084, 5.79) -> (74.0084, 5.79)
  line L104 (98.0084, 5.79) -> (74.0084, 5.79)
  line L105 (74.0084, 20.79) -> (98.0084, 20.79)
  line L106 (74.0084, 22.06) -> (98.0084, 22.06)
  line L107 (74.0084, 25.235) -> (98.0084, 25.235)
  line L108 (-48.0922, 0) -> (59.2659, 0) construction
  line L109 (-97.975, -56.35) -> (-73.975, -56.35)
  line L110 (-70.975, -53.35) -> (-70.975, -44.35)
  line L111 (-100.975, -44.35) -> (-100.975, -53.35)
  line L112 (-73.975, -41.35) -> (-97.975, -41.35)
  arc A100 (-100.975, -53.35) -> (-97.975, -56.35) centre (-97.975, -53.35) ccw
  arc A101 (-102.245, -53.35) -> (-97.975, -57.62) centre (-97.975, -53.35) ccw
  arc A102 (-97.975, -41.35) -> (-100.975, -44.35) centre (-97.975, -44.35) ccw
  arc A103 (-97.975, -40.08) -> (-102.245, -44.35) centre (-97.975, -44.35) ccw
  arc A104 (-97.975, -36.905) -> (-105.42, -44.35) centre (-97.975, -44.35) ccw
  line L113 (-100.975, -44.35) -> (-100.975, -53.35)
  arc A105 (-105.42, -53.35) -> (-97.975, -60.795) centre (-97.975, -53.35) ccw
  line L114 (-105.42, -44.35) -> (-105.42, -53.35)
  line L115 (-102.245, -44.35) -> (-102.245, -53.35)
  line L116 (-73.975, -40.08) -> (-97.975, -40.08)
  line L117 (-97.975, -60.795) -> (-73.975, -60.795)
  line L118 (-97.975, -56.35) -> (-73.975, -56.35)
  line L119 (-97.975, -57.62) -> (-73.975, -57.62)
  line L120 (-73.975, -41.35) -> (-97.975, -41.35)
  line L121 (-73.975, -41.35) -> (-97.975, -41.35)
  line L122 (-66.53, -53.35) -> (-66.53, -44.35)
  line L123 (-69.705, -53.35) -> (-69.705, -44.35)
  line L124 (-70.975, -53.35) -> (-70.975, -44.35)
  arc A106 (-66.53, -44.35) -> (-73.975, -36.905) centre (-73.975, -44.35) ccw
  arc A107 (-69.705, -44.35) -> (-73.975, -40.08) centre (-73.975, -44.35) ccw
  arc A108 (-70.975, -44.35) -> (-73.975, -41.35) centre (-73.975, -44.35) ccw
  arc A109 (-73.975, -56.35) -> (-70.975, -53.35) centre (-73.975, -53.35) ccw
  arc A110 (-73.975, -60.795) -> (-66.53, -53.35) centre (-73.975, -53.35) ccw
  arc A111 (-73.975, -57.62) -> (-69.705, -53.35) centre (-73.975, -53.35) ccw
  line L125 (-73.975, -36.905) -> (-97.975, -36.905)
  arc A112 (-73.975, -56.35) -> (-70.975, -53.35) centre (-73.975, -53.35) ccw
  arc A113 (-100.975, -53.35) -> (-97.975, -56.35) centre (-97.975, -53.35) ccw
  arc A114 (-97.975, -41.35) -> (-100.975, -44.35) centre (-97.975, -44.35) ccw
  arc A115 (-70.975, -44.35) -> (-73.975, -41.35) centre (-73.975, -44.35) ccw
  arc A116 (-13.6472, -44.35) -> (-16.6472, -41.35) centre (-16.6472, -44.35) ccw
  arc A117 (-12.3772, -44.35) -> (-16.6472, -40.08) centre (-16.6472, -44.35) ccw
  arc A118 (-9.2022, -44.35) -> (-16.6472, -36.905) centre (-16.6472, -44.35) ccw
  arc A119 (-40.6472, -40.08) -> (-44.9172, -44.35) centre (-40.6472, -44.35) ccw
  arc A120 (-40.6472, -36.905) -> (-48.0922, -44.35) centre (-40.6472, -44.35) ccw
  line L126 (-13.6472, -53.35) -> (-13.6472, -44.35)
  line L127 (-12.3772, -53.35) -> (-12.3772, -44.35)
  line L128 (-9.2022, -53.35) -> (-9.2022, -44.35)
  arc A121 (-16.6472, -56.35) -> (-13.6472, -53.35) centre (-16.6472, -53.35) ccw
  arc A122 (-16.6472, -57.62) -> (-12.3772, -53.35) centre (-16.6472, -53.35) ccw
  arc A123 (-16.6472, -60.795) -> (-9.2022, -53.35) centre (-16.6472, -53.35) ccw
  arc A124 (-43.6472, -53.35) -> (-40.6472, -56.35) centre (-40.6472, -53.35) ccw
  arc A125 (-40.6472, -41.35) -> (-43.6472, -44.35) centre (-40.6472, -44.35) ccw
  line L129 (-43.6472, -44.35) -> (-43.6472, -53.35)
  line L130 (-48.0922, -44.35) -> (-48.0922, -53.35)
  line L131 (-44.9172, -44.35) -> (-44.9172, -53.35)
  arc A126 (-48.0922, -53.35) -> (-40.6472, -60.795) centre (-40.6472, -53.35) ccw
  arc A127 (-44.9172, -53.35) -> (-40.6472, -57.62) centre (-40.6472, -53.35) ccw
  line L132 (-16.6472, -36.905) -> (-40.6472, -36.905)
  line L133 (-16.6472, -40.08) -> (-40.6472, -40.08)
  line L134 (-16.6472, -41.35) -> (-40.6472, -41.35)
  line L135 (-16.6472, -41.35) -> (-40.6472, -41.35)
  line L136 (-40.6472, -56.35) -> (-16.6472, -56.35)
  line L137 (-40.6472, -57.62) -> (-16.6472, -57.62)
  line L138 (-40.6472, -60.795) -> (-16.6472, -60.795)
  arc A128 (43.6806, -44.35) -> (40.6806, -41.35) centre (40.6806, -44.35) ccw
  arc A129 (44.9506, -44.35) -> (40.6806, -40.08) centre (40.6806, -44.35) ccw
  arc A130 (48.1256, -44.35) -> (40.6806, -36.905) centre (40.6806, -44.35) ccw
  arc A131 (16.6806, -40.08) -> (12.4106, -44.35) centre (16.6806, -44.35) ccw
  arc A132 (16.6806, -36.905) -> (9.2356, -44.35) centre (16.6806, -44.35) ccw
  line L139 (43.6806, -53.35) -> (43.6806, -44.35)
  line L140 (44.9506, -53.35) -> (44.9506, -44.35)
  line L141 (48.1256, -53.35) -> (48.1256, -44.35)
  arc A133 (40.6806, -56.35) -> (43.6806, -53.35) centre (40.6806, -53.35) ccw
  arc A134 (40.6806, -57.62) -> (44.9506, -53.35) centre (40.6806, -53.35) ccw
  arc A135 (40.6806, -60.795) -> (48.1256, -53.35) centre (40.6806, -53.35) ccw
  arc A136 (13.6806, -53.35) -> (16.6806, -56.35) centre (16.6806, -53.35) ccw
  arc A137 (16.6806, -41.35) -> (13.6806, -44.35) centre (16.6806, -44.35) ccw
  line L142 (13.6806, -44.35) -> (13.6806, -53.35)
  line L143 (9.2356, -44.35) -> (9.2356, -53.35)
  line L144 (12.4106, -44.35) -> (12.4106, -53.35)
  arc A138 (9.2356, -53.35) -> (16.6806, -60.795) centre (16.6806, -53.35) ccw
  arc A139 (12.4106, -53.35) -> (16.6806, -57.62) centre (16.6806, -53.35) ccw
  line L145 (40.6806, -36.905) -> (16.6806, -36.905)
  line L146 (40.6806, -40.08) -> (16.6806, -40.08)
  line L147 (40.6806, -41.35) -> (16.6806, -41.35)
  line L148 (40.6806, -41.35) -> (16.6806, -41.35)
  line L149 (16.6806, -56.35) -> (40.6806, -56.35)
  line L150 (16.6806, -57.62) -> (40.6806, -57.62)
  line L151 (16.6806, -60.795) -> (40.6806, -60.795)
  arc A140 (101.0084, -44.35) -> (98.0084, -41.35) centre (98.0084, -44.35) ccw
  arc A141 (102.2784, -44.35) -> (98.0084, -40.08) centre (98.0084, -44.35) ccw
  arc A142 (105.4534, -44.35) -> (98.0084, -36.905) centre (98.0084, -44.35) ccw
  arc A143 (74.0084, -40.08) -> (69.7384, -44.35) centre (74.0084, -44.35) ccw
  arc A144 (74.0084, -36.905) -> (66.5634, -44.35) centre (74.0084, -44.35) ccw
  line L152 (101.0084, -53.35) -> (101.0084, -44.35)
  line L153 (102.2784, -53.35) -> (102.2784, -44.35)
  line L154 (105.4534, -53.35) -> (105.4534, -44.35)
  arc A145 (98.0084, -56.35) -> (101.0084, -53.35) centre (98.0084, -53.35) ccw
  arc A146 (98.0084, -57.62) -> (102.2784, -53.35) centre (98.0084, -53.35) ccw
  arc A147 (98.0084, -60.795) -> (105.4534, -53.35) centre (98.0084, -53.35) ccw
  arc A148 (71.0084, -53.35) -> (74.0084, -56.35) centre (74.0084, -53.35) ccw
  arc A149 (74.0084, -41.35) -> (71.0084, -44.35) centre (74.0084, -44.35) ccw
  line L155 (71.0084, -44.35) -> (71.0084, -53.35)
  line L156 (66.5634, -44.35) -> (66.5634, -53.35)
  line L157 (69.7384, -44.35) -> (69.7384, -53.35)
  arc A150 (66.5634, -53.35) -> (74.0084, -60.795) centre (74.0084, -53.35) ccw
  arc A151 (69.7384, -53.35) -> (74.0084, -57.62) centre (74.0084, -53.35) ccw
  line L158 (98.0084, -36.905) -> (74.0084, -36.905)
  line L159 (98.0084, -40.08) -> (74.0084, -40.08)
  line L160 (98.0084, -41.35) -> (74.0084, -41.35)
  line L161 (98.0084, -41.35) -> (74.0084, -41.35)
  line L162 (74.0084, -56.35) -> (98.0084, -56.35)
  line L163 (74.0084, -57.62) -> (98.0084, -57.62)
  line L164 (74.0084, -60.795) -> (98.0084, -60.795)
  arc A152 (-70.975, -8.79) -> (-73.975, -5.79) centre (-73.975, -8.79) ccw
  arc A153 (-69.705, -8.79) -> (-73.975, -4.52) centre (-73.975, -8.79) ccw
  arc A154 (-66.53, -8.79) -> (-73.975, -1.345) centre (-73.975, -8.79) ccw
  arc A155 (-97.975, -4.52) -> (-102.245, -8.79) centre (-97.975, -8.79) ccw
  arc A156 (-97.975, -1.345) -> (-105.42, -8.79) centre (-97.975, -8.79) ccw
  line L165 (-70.975, -17.79) -> (-70.975, -8.79)
  line L166 (-69.705, -17.79) -> (-69.705, -8.79)
  line L167 (-66.53, -17.79) -> (-66.53, -8.79)
  arc A157 (-73.975, -20.79) -> (-70.975, -17.79) centre (-73.975, -17.79) ccw
  arc A158 (-73.975, -22.06) -> (-69.705, -17.79) centre (-73.975, -17.79) ccw
  arc A159 (-73.975, -25.235) -> (-66.53, -17.79) centre (-73.975, -17.79) ccw
  arc A160 (-100.975, -17.79) -> (-97.975, -20.79) centre (-97.975, -17.79) ccw
  arc A161 (-97.975, -5.79) -> (-100.975, -8.79) centre (-97.975, -8.79) ccw
  line L168 (-100.975, -8.79) -> (-100.975, -17.79)
  line L169 (-105.42, -8.79) -> (-105.42, -17.79)
  line L170 (-102.245, -8.79) -> (-102.245, -17.79)
  arc A162 (-105.42, -17.79) -> (-97.975, -25.235) centre (-97.975, -17.79) ccw
  arc A163 (-102.245, -17.79) -> (-97.975, -22.06) centre (-97.975, -17.79) ccw
  line L171 (-73.975, -1.345) -> (-97.975, -1.345)
  line L172 (-73.975, -4.52) -> (-97.975, -4.52)
  line L173 (-73.975, -5.79) -> (-97.975, -5.79)
  line L174 (-73.975, -5.79) -> (-97.975, -5.79)
  line L175 (-97.975, -20.79) -> (-73.975, -20.79)
  line L176 (-97.975, -22.06) -> (-73.975, -22.06)
  line L177 (-97.975, -25.235) -> (-73.975, -25.235)
  arc A164 (-13.6472, -8.79) -> (-16.6472, -5.79) centre (-16.6472, -8.79) ccw
  arc A165 (-12.3772, -8.79) -> (-16.6472, -4.52) centre (-16.6472, -8.79) ccw
  arc A166 (-9.2022, -8.79) -> (-16.6472, -1.345) centre (-16.6472, -8.79) ccw
  arc A167 (-40.6472, -4.52) -> (-44.9172, -8.79) centre (-40.6472, -8.79) ccw
  arc A168 (-40.6472, -1.345) -> (-48.0922, -8.79) centre (-40.6472, -8.79) ccw
  line L178 (-13.6472, -17.79) -> (-13.6472, -8.79)
  line L179 (-12.3772, -17.79) -> (-12.3772, -8.79)
  line L180 (-9.2022, -17.79) -> (-9.2022, -8.79)
  arc A169 (-16.6472, -20.79) -> (-13.6472, -17.79) centre (-16.6472, -17.79) ccw
  arc A170 (-16.6472, -22.06) -> (-12.3772, -17.79) centre (-16.6472, -17.79) ccw
  arc A171 (-16.6472, -25.235) -> (-9.2022, -17.79) centre (-16.6472, -17.79) ccw
  arc A172 (-43.6472, -17.79) -> (-40.6472, -20.79) centre (-40.6472, -17.79) ccw
  arc A173 (-40.6472, -5.79) -> (-43.6472, -8.79) centre (-40.6472, -8.79) ccw
  line L181 (-43.6472, -8.79) -> (-43.6472, -17.79)
  line L182 (-48.0922, -8.79) -> (-48.0922, -17.79)
  line L183 (-44.9172, -8.79) -> (-44.9172, -17.79)
  arc A174 (-48.0922, -17.79) -> (-40.6472, -25.235) centre (-40.6472, -17.79) ccw
  arc A175 (-44.9172, -17.79) -> (-40.6472, -22.06) centre (-40.6472, -17.79) ccw
  line L184 (-16.6472, -1.345) -> (-40.6472, -1.345)
  line L185 (-16.6472, -4.52) -> (-40.6472, -4.52)
  line L186 (-16.6472, -5.79) -> (-40.6472, -5.79)
  line L187 (-16.6472, -5.79) -> (-40.6472, -5.79)
  line L188 (-40.6472, -20.79) -> (-16.6472, -20.79)
  line L189 (-40.6472, -22.06) -> (-16.6472, -22.06)
  line L190 (-40.6472, -25.235) -> (-16.6472, -25.235)
  arc A176 (43.6806, -8.79) -> (40.6806, -5.79) centre (40.6806, -8.79) ccw
  arc A177 (44.9506, -8.79) -> (40.6806, -4.52) centre (40.6806, -8.79) ccw
  arc A178 (48.1256, -8.79) -> (40.6806, -1.345) centre (40.6806, -8.79) ccw
  arc A179 (16.6806, -4.52) -> (12.4106, -8.79) centre (16.6806, -8.79) ccw
  arc A180 (16.6806, -1.345) -> (9.2356, -8.79) centre (16.6806, -8.79) ccw
  line L191 (43.6806, -17.79) -> (43.6806, -8.79)
  line L192 (44.9506, -17.79) -> (44.9506, -8.79)
  line L193 (48.1256, -17.79) -> (48.1256, -8.79)
  arc A181 (40.6806, -20.79) -> (43.6806, -17.79) centre (40.6806, -17.79) ccw
  arc A182 (40.6806, -22.06) -> (44.9506, -17.79) centre (40.6806, -17.79) ccw
  arc A183 (40.6806, -25.235) -> (48.1256, -17.79) centre (40.6806, -17.79) ccw
  arc A184 (13.6806, -17.79) -> (16.6806, -20.79) centre (16.6806, -17.79) ccw
  arc A185 (16.6806, -5.79) -> (13.6806, -8.79) centre (16.6806, -8.79) ccw
  line L194 (13.6806, -8.79) -> (13.6806, -17.79)
  line L195 (9.2356, -8.79) -> (9.2356, -17.79)
  line L196 (12.4106, -8.79) -> (12.4106, -17.79)
  arc A186 (9.2356, -17.79) -> (16.6806, -25.235) centre (16.6806, -17.79) ccw
  arc A187 (12.4106, -17.79) -> (16.6806, -22.06) centre (16.6806, -17.79) ccw
  line L197 (40.6806, -1.345) -> (16.6806, -1.345)
  line L198 (40.6806, -4.52) -> (16.6806, -4.52)
  line L199 (40.6806, -5.79) -> (16.6806, -5.79)
  line L200 (40.6806, -5.79) -> (16.6806, -5.79)
  line L201 (16.6806, -20.79) -> (40.6806, -20.79)
  line L202 (16.6806, -22.06) -> (40.6806, -22.06)
  line L203 (16.6806, -25.235) -> (40.6806, -25.235)
  arc A188 (101.0084, -8.79) -> (98.0084, -5.79) centre (98.0084, -8.79) ccw
  arc A189 (102.2784, -8.79) -> (98.0084, -4.52) centre (98.0084, -8.79) ccw
  arc A190 (105.4534, -8.79) -> (98.0084, -1.345) centre (98.0084, -8.79) ccw
  arc A191 (74.0084, -4.52) -> (69.7384, -8.79) centre (74.0084, -8.79) ccw
  arc A192 (74.0084, -1.345) -> (66.5634, -8.79) centre (74.0084, -8.79) ccw
  line L204 (101.0084, -17.79) -> (101.0084, -8.79)
  line L205 (102.2784, -17.79) -> (102.2784, -8.79)
  line L206 (105.4534, -17.79) -> (105.4534, -8.79)
  arc A193 (98.0084, -20.79) -> (101.0084, -17.79) centre (98.0084, -17.79) ccw
  arc A194 (98.0084, -22.06) -> (102.2784, -17.79) centre (98.0084, -17.79) ccw
  arc A195 (98.0084, -25.235) -> (105.4534, -17.79) centre (98.0084, -17.79) ccw
  arc A196 (71.0084, -17.79) -> (74.0084, -20.79) centre (74.0084, -17.79) ccw
  arc A197 (74.0084, -5.79) -> (71.0084, -8.79) centre (74.0084, -8.79) ccw
  line L207 (71.0084, -8.79) -> (71.0084, -17.79)
  line L208 (66.5634, -8.79) -> (66.5634, -17.79)
  line L209 (69.7384, -8.79) -> (69.7384, -17.79)
  arc A198 (66.5634, -17.79) -> (74.0084, -25.235) centre (74.0084, -17.79) ccw
  arc A199 (69.7384, -17.79) -> (74.0084, -22.06) centre (74.0084, -17.79) ccw
  line L210 (98.0084, -1.345) -> (74.0084, -1.345)
  line L211 (98.0084, -4.52) -> (74.0084, -4.52)
  line L212 (98.0084, -5.79) -> (74.0084, -5.79)
  line L213 (98.0084, -5.79) -> (74.0084, -5.79)
  line L214 (74.0084, -20.79) -> (98.0084, -20.79)
  line L215 (74.0084, -22.06) -> (98.0084, -22.06)
  line L216 (74.0084, -25.235) -> (98.0084, -25.235)
  point P0 (0, 0)
  dimension "d453" = 1.27
  dimension "d454" = 1.27
  dimension "d455" = 1.27
  dimension "d456" = 1.27
  dimension "d457" = 3.175
  dimension "d458" = 3.175
  dimension "d459" = 3.175
  dimension "d460" = 3.175
  dimension "d470" = 57.3278
  dimension "d473" = 35.56
  constraints: 442 end point, 392 point on circle, 294 symmetric about line, 196 centre point, 130 coincident, 8 horizontal alignment, 8 vertical alignment, 4 concentric, 3 collinear, 2 horizontal, 1 vertical, 526 other
  measures "d453" radial gap between concentric circles of A1 A0
  measures "d454" radial gap between concentric circles of A5 A2
  measures "d455" radial gap between concentric circles of A3 A6
  measures "d456" radial gap between concentric circles of A7 A4
  measures "d457" radial gap between concentric circles of A8 A1
  measures "d458" radial gap between concentric circles of A9 A5
  measures "d459" radial gap between concentric circles of A6 A10
  measures "d460" radial gap between concentric circles of A11 A7
  measures "d470" distance of L9.end L18.end
  measures "d473" distance of L9.end L57.end
extrude "Extrusion9" cut sketch "Seal Seating" against normal blind 2.3813 contours L14 A9 L15 A10 L16 A11 L13 A8 | L23 A20 L21 A26 L29 A23 L19 A18 | L36 A32 L34 A38 L42 A35 L32 A30 | L49 A44 L47 A50 L55 A47 L45 A42 | L62 A56 L60 A62 L68 A59 L58 A54 | L75 A68 L73 A74 L81 A71 L71 A66 | L88 A80 L86 A86 L94 A83 L84 A78 | L101 A92 L99 A98 L107 A95 L97 A90 | L125 A106 L122 A110 L117 A105 L114 A104 | L128 A123 L138 A126 L130 A120 L132 A118 | L141 A135 L151 A138 L143 A132 L145 A130 | L154 A147 L164 A150 L156 A144 L158 A142 | L167 A159 L177 A162 L169 A156 L171 A154 | L180 A171 L190 A174 L182 A168 L184 A166 | L193 A183 L203 A186 L195 A180 L197 A178 | L206 A195 L216 A198 L208 A192 L210 A190
equation "\"d328\" = d286"
